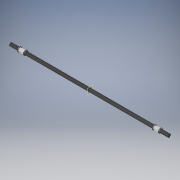
# Autodesk Inventor part: roller-stick-v2
Saved by Autodesk Inventor 2019 (Build 230136000, 136)
## iProperties
Created: 2019-04-14
Part Number: roller-stick-v2
Material: Generic
Document SubType Name: Modeling
Designer: Tesler
Density: 1 g/cm^3
Appearance: Default
Author: Tesler
Autodesk Inventor part; units mm, degrees
sketch "Sketch1" plane through (0, 0, 0) normal (1, 0, 0) x (0, 1, 0)
  arc A0 (-0.4, -2.25) -> (-2.1861, -0.5323) centre (-2.1497, -2.2819) ccw
  arc A1 (2.1843, -0.5396) -> (0.4, -2.25) centre (2.1496, -2.2892) ccw
  arc A2 (0.4, 2.25) -> (2.1843, 0.5396) centre (2.1496, 2.2892) ccw
  arc A3 (-2.1861, 0.5323) -> (-0.4, 2.25) centre (-2.1497, 2.2819) ccw
  arc A4 (-2.1861, 0.5323) -> (-2.1861, -0.5323) centre (0, 0) ccw
  arc A5 (2.1843, -0.5396) -> (2.1843, 0.5396) centre (0, 0) ccw
  line L0 (-0.4, 2.25) -> (0.4, 2.25)
  line L1 (-0.4, -2.25) -> (0.4, -2.25)
  point P0 (0, 0)
  point P1 (0, 0)
  point P2 (2.1843, -0.5396)
  dimension "d3" = 1.75
  dimension "d4" = 1.75
  dimension "d5" = 2.25
  dimension "d10" = 4.3705
  dimension "d12" = 1.7844
  dimension "d13" = 1.7861
  dimension "d14" = 1.7104
  dimension "d15" = 27.368
  dimension "d16" = 76.125
  dimension "d17" = 2.25
  dimension "d18" = 1.75
  dimension "d19" = 1.75
  dimension "d20" = 4.5
  dimension "d21" = 2.7896
  dimension "d22" = 1.7177
  dimension "d23" = 2.7823
  dimension "d24" = 2.5861
  dimension "d25" = 2.7753
  dimension "d26" = 2.7753
  constraints: 12 point on circle, 6 centre point, 4 end point, 2 horizontal
  measures "d3" radius of A0
  measures "d4" radius of A1
  measures "d5" radius of A4
  measures "d10" distance of point (2.184, -0.54) A0.end
  measures "d12" horizontal distance of A1.start L1.end
  measures "d13" horizontal distance of L0.start A4.start
  measures "d14" vertical distance of A5.end L0.end
  measures "d17" radius of A5
  measures "d18" radius of A2
  measures "d19" radius of A3
  measures "d20" distance between parallel lines of L1 L0
  measures "d21" distance from line of L0 A1.start
  measures "d22" vertical distance of A4.start L0.start
  measures "d23" distance from line of A0.end L0
  measures "d24" horizontal distance of A4.start L0.end
extrude "Extrusion1" add sketch "Sketch1" along normal blind 204.3792
fillet "Fillet1" radius 0.3 16 edges at (204.3792, 0.9386, 1.0259) (204.3792, 2.25, 0) (204.3792, 0.9386, -1.0259) (204.3792, 0, -2.25) (204.3792, -0.9367, -1.0205) (204.3792, -2.25, 0) (204.3792, -0.9367, 1.0205) (204.3792, 0, 2.25) (0, 2.25, 0) (0, 0.9386, 1.0259) (0, 0, 2.25) (0, 0.9386, -1.0259) (0, 0, -2.25) (0, -0.9367, -1.0205) (0, -0.9367, 1.0205) (0, -2.25, 0)
sketch "Sketch2" plane through (0, 0, 0) normal (-1, 0, 0) x (0, 0, 1)
  circle A0 centre (0, 0) radius 0.75
  dimension "d30" = 1.5
  constraints: 1 centre point, 1 coincident
  measures "d30" diameter of A0
extrude "Extrusion2" add sketch "Sketch2" along normal blind 0.15
ref_plane "Work Plane1" through (102.1896, 0, 0) normal (-1, 0, 0) x (0, 0, 1)
mirror "Mirror1" about plane through (102.1896, 0, 0) normal (-1, 0, 0) of "Extrusion2"
ref_plane "Work Plane2" through (10.9625, 0, 0) normal (-1, 0, 0) x (0, 0, 1)
sketch "Sketch3" plane through (10.9625, 0, 0) normal (-1, 0, 0) x (0, 0, 1)
  circle A0 centre (0, 0) radius 1.1
  circle A1 centre (0, 0) radius 3
  point P0 (2.25, 0.4)
  dimension "d34" = 2.2
  dimension "d35" = 6
  constraints: 2 centre point, 2 coincident
  measures "d34" diameter of A0
  measures "d35" diameter of A1
extrude "Extrusion3" add sketch "Sketch3" against normal blind 0.7937
ref_plane "Work Plane3" through (11.7563, 0, 0) normal (1, 0, 0) x (0, 0, -1)
sketch "Sketch4" plane through (11.7563, 0, 0) normal (1, 0, 0) x (0, 0, -1)
  circle A0 centre (0, 0) radius 1.1
  line L0 (2.25, 0.4) -> (2.25, -0.4) projected
  circle A1 centre (0, 0) radius 2.2853
  dimension "d39" = 2.2
  constraints: 2 coincident, 1 centre point, 3 other
  measures "d39" diameter of A0
extrude "Extrusion4" add sketch "Sketch4" along normal blind 7.1437
sketch "Sketch5" plane through (18.9, 0, 0) normal (1, 0, 0) x (0, 0, -1)
  circle A0 centre (0, 0) radius 1.1
  circle A1 centre (0, 0) radius 3
  dimension "d42" = 6
  dimension "d43" = 2.2
  constraints: 2 centre point, 2 coincident
  measures "d42" diameter of A1
  measures "d43" diameter of A0
extrude "Extrusion5" add sketch "Sketch5" along normal blind 0.7937
sketch "Sketch6" plane through (10.9625, 0, 0) normal (-1, 0, 0) x (0, 0, 1)
  arc A0 (0.5396, 2.1843) -> (2.25, 0.4) centre (2.2892, 2.1496) ccw projected
  arc A1 (0.5396, 2.1843) -> (-0.5396, 2.1843) centre (0, 0) ccw projected
  line L0 (2.25, -0.4) -> (2.25, 0.4) projected
  arc A2 (2.25, -0.4) -> (0.5323, -2.1861) centre (2.2819, -2.1497) ccw projected
  arc A3 (-0.5323, -2.1861) -> (0.5323, -2.1861) centre (0, 0) ccw projected
  arc A4 (-0.5323, -2.1861) -> (-2.25, -0.4) centre (-2.2819, -2.1497) ccw projected
  line L1 (-2.25, 0.4) -> (-2.25, -0.4) projected
  arc A5 (-2.25, 0.4) -> (-0.5396, 2.1843) centre (-2.2892, 2.1496) ccw projected
  circle A6 centre (0, 0) radius 2.2853 projected
  circle A7 centre (0, 0) radius 2.2853
  arc A8 (0.5396, 2.1843) -> (2.25, 0.4) centre (2.2892, 2.1496) ccw projected
  arc A9 (0.5396, 2.1843) -> (2.25, 0.4) centre (2.2892, 2.1496) ccw
  arc A10 (2.25, -0.4) -> (0.5323, -2.1861) centre (2.2819, -2.1497) ccw projected
  arc A11 (2.25, -0.4) -> (0.5323, -2.1861) centre (2.2819, -2.1497) ccw
  line L2 (2.25, 0.4) -> (2.25, -0.4)
  line L3 (-2.25, -0.4) -> (-2.25, 0.4) projected
  line L4 (-2.25, 0.4) -> (-2.25, -0.4)
  arc A12 (-0.5323, -2.1861) -> (-2.25, -0.4) centre (-2.2819, -2.1497) ccw projected
  arc A13 (-0.5323, -2.1861) -> (-2.25, -0.4) centre (-2.2819, -2.1497) ccw
  arc A14 (-0.5323, -2.1861) -> (0.5323, -2.1861) centre (0, 0) ccw projected
  arc A15 (-0.5323, -2.1861) -> (0.5323, -2.1861) centre (0, 0) ccw
  arc A16 (-2.25, 0.4) -> (-0.5396, 2.1843) centre (-2.2892, 2.1496) ccw projected
  arc A17 (-2.25, 0.4) -> (-0.5396, 2.1843) centre (-2.2892, 2.1496) ccw
  arc A18 (0.5396, 2.1843) -> (-0.5396, 2.1843) centre (0, 0) ccw
  constraints: 12 point on circle, 7 centre point, 4 end point, 3 concentric, 1 coincident, 1 collinear, 1 vertical
extrude "Extrusion6" cut sketch "Sketch6" against normal blind 0.1
ref_plane "Work Plane4" through (15.3281, 0, 0) normal (1, 0, 0) x (0, 0, -1)
mirror "Mirror2" about plane through (15.3281, 0, 0) normal (1, 0, 0) of "Extrusion6"
fillet "Fillet2" radius 0.3 6 edges at (11.7563, 0, -3) (10.9625, 0, -3) (11.7563, 0, 2.2853) (18.9, 0, 3) (18.9, 0, 2.2853) (19.6938, 0, 3)
ref_plane "Work Plane5" through (102.1896, 0, 0) normal (-1, 0, 0) x (0, 0, 1)
mirror "Mirror3" about plane through (102.1896, 0, 0) normal (-1, 0, 0) of "Fillet2", "Extrusion4", "Extrusion5", "Extrusion3"
body "Solid1"
